Autodesk Fusion 360 part; units mm, degrees
(part 2 of 2)
sketch "Sketch7" plane through (0, 0, 1.6) normal (0, 0, -1) x (1, 0, 0)
  line L0 (96, 57.5) -> (-16, 57.5)
  line L1 (-20, 53.5) -> (-20, -23.5)
  line L2 (-16, -27.5) -> (96, -27.5)
  line L3 (100, -23.5) -> (100, 53.5)
  line L4 (40, 57.5) -> (40, -27.5) construction
  line L5 (100, 15) -> (-20, 15) construction
  line L6 (91, -22.5) -> (-11, -22.5)
  line L7 (-15, -18.5) -> (-15, 48.5)
  line L8 (-11, 52.5) -> (91, 52.5)
  line L9 (95, 48.5) -> (95, -18.5)
  line L10 (95, -22.5) -> (-15, 52.5) construction
  line L11 (-15, -22.5) -> (95, 52.5) construction
  arc A0 (-16, 57.5) -> (-20, 53.5) centre (-16, 53.5) ccw
  arc A1 (-20, -23.5) -> (-16, -27.5) centre (-16, -23.5) ccw
  arc A2 (96, -27.5) -> (100, -23.5) centre (96, -23.5) ccw
  arc A3 (100, 53.5) -> (96, 57.5) centre (96, 53.5) ccw
  arc A4 (-11, 52.5) -> (-15, 48.5) centre (-11, 48.5) ccw
  arc A5 (95, 48.5) -> (91, 52.5) centre (91, 48.5) ccw
  arc A6 (91, -22.5) -> (95, -18.5) centre (91, -18.5) ccw
  arc A7 (-15, -18.5) -> (-11, -22.5) centre (-11, -18.5) ccw
  point P0 (40, 15)
  dimension "d62" = 110
  dimension "d65" = 75
  dimension "d72" = 4
  dimension "d73" = 4
  dimension "d74" = 4
  dimension "d75" = 4
  constraint midpoint L0 L4.start
  constraint midpoint L2 L4.end
  constraint midpoint L3 L5.start
  constraint midpoint L1 L5.end
  constraint horizontal L6
  constraint perpendicular L6 L7
  constraint parallel L6 L8
  constraint parallel L7 L9
  constraint coincident L10 P0
  constraint coincident L11 P0
  constraint midpoint L4 P0
  constraint coincident L10.end L8
  constraint coincident L10.end L7
  constraint tangent L8 A4
  constraint tangent L7 A4
  constraint coincident L11.end L9
  constraint coincident L11.end L8
  constraint tangent L9 A5
  constraint tangent L8 A5
  constraint coincident L10.start L9
  constraint coincident L10.start L6
  constraint tangent L9 A6
  constraint tangent L6 A6
  constraint coincident L11.start L6
  constraint coincident L11.start L7
  constraint tangent L6 A7
  constraint tangent L7 A7
  measures "d62" distance of L10.end L11.end
  measures "d65" distance of L11.start L10.end
  measures "d72" radius of A4
  measures "d73" radius of A5
  measures "d74" radius of A6
  measures "d75" radius of A7
extrude "Extrude9" cut sketch "Sketch7" against normal blind 8.4 contours L6 L7 L8 L9 A4 A5 A6 A7
equation "ORingDiameter = 1.78 mm" comment "Diamter of the O ring"
equation "ORingInnerDiameter = 170 mm" comment "Inner diamter of the o ring bore"
equation "d25 = ( ORingPerimeter - 100 mm ) / 4 + 50 mm"
equation "ORingPerimeter = 2 * 3.1412 * ( ( ORingInnerDiameter / 2 ) + ORingDiameter / 2 )"
equation "d27 = ( ORingPerimeter - 100 mm ) / 4"
equation "d28 = ( ( ORingDiameter * 1.05 ) / 2 ) + 0.5 mm"
equation "d29 = ( ( ORingDiameter * 1.05 ) / 2 ) + 0.5 mm"
equation "d30 = ( ( ORingDiameter * 1.05 ) / 2 ) + 0.5 mm"
equation "d31 = ( ( ORingDiameter * 1.05 ) / 2 ) + 0.5 mm"
equation "d32 = ORingDiameter * 0.8"
equation "d36 = ( ORingPerimeter - 100 mm ) / 4 + 50 mm"
equation "d37 = ( ORingPerimeter - 100 mm ) / 4"
equation "d38 = ( ORingDiameter * 1.05 ) / 2"
equation "d39 = ( ORingDiameter * 1.05 ) / 2"
equation "d40 = ( ORingDiameter * 1.05 ) / 2"
equation "d41 = ( ORingDiameter * 1.05 ) / 2"
equation "d44 = ( ORingDiameter ) * 6 + ORingDiameter * 0.05 - 0.5 mm"
equation "d45 = ( ORingDiameter ) * 6 + ( ORingDiameter * 1.1 ) + 0.5 mm"
equation "d50 = ( ORingDiameter ) * 6 + ORingDiameter * 0.05 - 0.0 mm"
equation "d51 = ( ORingDiameter ) * 6 + ORingDiameter * 1.1 + 0 mm"
equation "d52 = -( ORingDiameter * 0.8 )"
equation "PanelWidth = 85 mm"
equation "PanelLength = 120 mm"
equation "d58 = PanelLength"
equation "d59 = PanelWidth"
equation "d62 = PanelLength - 10 mm"
equation "d65 = PanelWidth - 10 mm"
